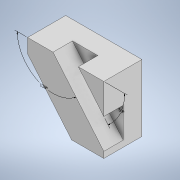
# Autodesk Inventor part: jjig02
Saved by Autodesk Inventor 2020.2 (Build 242310000, 310)
## iProperties
Created: 2020-02-27
Part Number: jjig02
Material: Generic
Document SubType Name: Modeling
Designer: robst
Density: 1 g/cm^3
Appearance: Default
Author: robst
Autodesk Inventor part; units mm, degrees
ref_plane "YZ Plane" through (0, 0, 0) normal (1, 0, 0) x (0, 1, 0)
ref_plane "XZ Plane" through (0, 0, 0) normal (0, 1, 0) x (-1, 0, 0)
ref_plane "XY Plane" through (0, 0, 0) normal (0, 0, 1) x (1, 0, 0)
sketch "Sketch1" plane through (0, 0, 0) normal (0, 0, 1) x (1, 0, 0)
  line L0 (-50.8, -44.45) -> (50.8, -44.45)
  line L1 (50.8, -44.45) -> (50.8, 44.45)
  line L2 (50.8, 44.45) -> (-50.8, 44.45)
  line L3 (-50.8, 44.45) -> (-50.8, -44.45)
  line L4 (-50.8, -44.45) -> (50.8, 44.45) construction
  line L5 (50.8, -44.45) -> (-50.8, 44.45) construction
  point P0 (0, 0)
  dimension "d0" = 101.6
  dimension "d1" = 88.9
  constraints: 12 end point, 2 midpoint, 2 parallel, 1 horizontal, 1 perpendicular
  measures "d0" distance of L0.start L0.end
  measures "d1" distance of L1.end L0.end
extrude "Extrusion1" add sketch "Sketch1" along normal blind 50.8
sketch "Sketch2" plane through (0, 0, 50.8) normal (0, 0, 1) x (1, 0, 0)
  line L0 (50.8, 44.45) -> (-50.8, 44.45) projected
  line L1 (0, 44.45) -> (50.8, -16.0911) construction
  line L2 (50.8, -44.45) -> (50.8, 44.45) projected
  line L3 (0, 44.45) -> (79.0308, 44.45) construction
  line L4 (16.9102, 44.45) -> (50.8, 4.0618)
  line L5 (-16.9102, 44.45) -> (50.8, -36.2439)
  line L6 (-16.9102, 44.45) -> (16.9102, 44.45)
  line L7 (50.8, 4.0618) -> (50.8, -36.2439)
  point P0 (0, 0)
  dimension "d4" = 50
  dimension "d5" = 12.954
  dimension "d15" = 12.954
  constraints: 12 end point, 5 point on line, 2 parallel, 1 collinear, 1 equal length, 1 horizontal, 1 midpoint
  measures "d4" angle of L1 L3
  measures "d5" distance between parallel lines of L4 L1
  measures "d15" distance between parallel lines of L5 L1
extrude "Extrusion2" cut sketch "Sketch2" against normal blind 25.908 contours L4 L2 L5 L0
sketch "Sketch3" plane through (0, 0, 50.8) normal (0, 0, 1) x (1, 0, 0)
  line L0 (50.8, -36.2439) -> (-16.9102, 44.45) projected
  line L1 (-50.8, 44.45) -> (-50.8, -44.45) projected
  line L2 (-50.8, 25.5652) -> (7.9497, -44.45)
  line L3 (-50.8, -44.45) -> (50.8, -44.45) projected
  line L4 (7.9497, -44.45) -> (-50.8, -44.45)
  line L5 (-50.8, -44.45) -> (-50.8, 25.5652)
  point P0 (0, 0)
  dimension "d16" = 38.1
  constraints: 6 end point, 2 point on line, 1 collinear, 1 parallel, 1 perpendicular
  measures "d16" distance between parallel lines of L2 L0
extrude "Extrusion3" cut sketch "Sketch3" against normal through all
equation "\"d5\" = 0.5 * widthFor1inch"
equation "\"d15\" = 0.5 * widthFor1inch"
equation "\"d7\" = widthFor1inch"
equation "\"widthFor1inch\" = 25.908"
body "Solid1"
